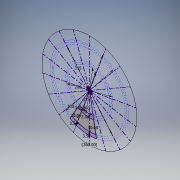
# Autodesk Inventor part: stator-bottom-connector
Saved by Autodesk Inventor 2018 (Build 220112000, 112)
## iProperties
Created: 2025-04-02
Part Number: stator-bottom-connector
Material: Generic
Document SubType Name: Modeling
Designer: neo
Density: 1 g/cm^3
Appearance: Default
Author: neo
Autodesk Inventor part; units mm, degrees
ref_plane "YZ Plane" through (0, 0, 0) normal (1, 0, 0) x (0, 1, 0)
ref_plane "XZ Plane" through (0, 0, 0) normal (0, 1, 0) x (-1, 0, 0)
ref_plane "XY Plane" through (0, 0, 0) normal (0, 0, 1) x (1, 0, 0)
sketch "Sketch1" plane through (0, 0, 0) normal (0, 1, 0) x (-1, 0, 0)
  circle A0 centre (0, 0) radius 89 construction
  circle A1 centre (0, 0) radius 104 construction
  circle A2 centre (0, 0) radius 157.5 construction
  circle A3 centre (0, 0) radius 172.5 construction
  circle A4 centre (0, 0) radius 96.5 construction
  circle A5 centre (0, 0) radius 165 construction
  line L0 (0, 0) -> (0, -209.0924)
  line L1 (0, 0) -> (71.5138, -196.4826)
  line L2 (0, 0) -> (134.402, -160.1741)
  line L3 (0, 0) -> (181.0793, -104.5462)
  line L4 (0, 0) -> (205.9158, -36.3085)
  line L5 (0, 0) -> (205.9158, 36.3085)
  line L6 (0, 0) -> (181.0793, 104.5462)
  line L7 (0, 0) -> (134.402, 160.1741)
  line L8 (0, 0) -> (71.5138, 196.4826)
  line L9 (0, 0) -> (0, 209.0924)
  line L10 (0, 0) -> (-71.5138, 196.4826)
  line L11 (0, 0) -> (-134.402, 160.1741)
  line L12 (0, 0) -> (-181.0793, 104.5462)
  line L13 (0, 0) -> (-205.9158, 36.3085)
  line L14 (0, 0) -> (-205.9158, -36.3085)
  line L15 (0, 0) -> (-181.0793, -104.5462)
  line L16 (0, 0) -> (-134.402, -160.1741)
  line L17 (0, 0) -> (-71.5138, -196.4826)
  circle A6 centre (33.0049, -90.6803) radius 1.75
  circle A7 centre (56.4333, -155.0493) radius 1.75
  circle A8 centre (0, -96.5) radius 1.75
  circle A9 centre (0, -165) radius 1.75
  line L18 (0, 0) -> (86.25, -149.3894)
  line L19 (0, 0) -> (-29.9543, -169.8793)
  arc A10 (-29.9543, -169.8793) -> (86.25, -149.3894) centre (0, 0) ccw
  arc A11 (-15.4547, -87.6479) -> (44.5, -77.0763) centre (0, 0) ccw
  arc A12 (-18.0594, -102.42) -> (52, -90.0666) centre (0, 0) ccw
  arc A13 (-27.3496, -155.1072) -> (78.75, -136.399) centre (0, 0) ccw
  dimension "d0" = 178
  dimension "d1" = 208
  dimension "d2" = 315
  dimension "d3" = 345
  dimension "d4" = 193
  dimension "d5" = 330
  dimension "d8" = 360
  dimension "d11" = 3.5
  dimension "d13" = 3.5
  dimension "d14" = 3.5
  dimension "d15" = 3.5
  dimension "d23" = 10
  dimension "d24" = 10
  constraints: 40 end point, 20 point on circle, 14 centre point, 10 coincident, 10 point on line, 1 vertical, 55 other
  measures "d0" diameter of A0
  measures "d1" diameter of A1
  measures "d2" diameter of A2
  measures "d3" diameter of A3
  measures "d4" diameter of A4
  measures "d5" diameter of A5
  measures "d11" diameter of A6
  measures "d13" diameter of A7
  measures "d14" diameter of A8
  measures "d15" diameter of A9
  measures "d23" angle of L1 L18
  measures "d24" angle of L19 L0
extrude "Extrusion1" add sketch "Sketch1" along normal blind 5 contours A11 L1 A6 A12 L0 A8 | L0 A8 A12 L19 A11 | A11 L18 A12 L1 A6 | L18 A10 L1 A7 A13 | A13 L0 A9 A10 L19 | L1 A7 A10 L0 A9 A13
extrude "Extrusion2" add sketch "Sketch1" along normal blind 2 contours L18 A13 L1 A12 | A12 L0 A13 L19 | L1 A13 L0 A12
chamfer "Chamfer1" distance 2 angle 45 4 edges at (1.75, 0, -96.5) (1.75, 0, -165) (-54.6833, 0, -155.0493) (-31.2549, 0, -90.6803)
body "Solid1"
